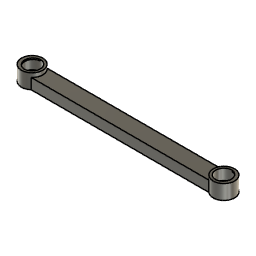
Sus_Arm_Prot_1 v1 (Autodesk Fusion 360 design; units mm, degrees)
Autodesk Fusion 360 part; units mm, degrees
sketch "Sketch1" plane through (0, 0, 0) normal (0, 0, 1) x (1, 0, 0)
  line L0 (0, 0) -> (32, 0)
  line L1 (32, 0) -> (32, -6)
  line L2 (32, -6) -> (0, -6)
  line L3 (0, -6) -> (0, 0)
  circle A0 centre (36.0053, -3) radius 4
  line L4 (32, 0) -> (33.3595, 0)
  line L5 (32, -6) -> (33.3595, -6)
  dimension "d1" = 32
  dimension "d2" = 6
  dimension "d3" = 8
  constraint horizontal L0
  constraint vertical L1
  constraint horizontal L2
  constraint vertical L3
  constraint coincident L0.start L3.end
  constraint coincident A0 L4.end
  constraint perpendicular L1 L4
  constraint coincident A0 L5.end
  constraint perpendicular L1 L5
  measures "d1" distance of L0.start L0.end
  measures "d2" distance of L0.start L2.end
  measures "d3" diameter of A0
extrude "Extrude1" add sketch "Sketch1" along normal blind 4 contours L0 L1 L2 L3 | L1 A0 L4 L5
extrude "Extrude2" add sketch "Sketch1" along normal blind 5.5 contours A0
hole "Hole1" at (36.0053, -3, 5.5) direction (0, 0, -1) diameter 6.2 depth 4 tip angle 180
sketch "Sketch2" plane through (0, 0, 5.5) normal (0, 0, 1) x (-1, 0, 0)
  circle A0 centre (-36.0053, 3) radius 3.1
  circle A1 centre (-36.0053, 3) radius 4
  arc A2 (-36.0053, 6.1) -> (-36.0053, -0.1) centre (-35.6842, 3) ccw
  constraint coincident A0 A2.start
  constraint coincident A0 A2.end
extrude "Extrude3" add sketch "Sketch2" against normal blind 0.5 contours A0 A2 picked at (-38.8883, 3.2291)
mirror "Mirror1" about plane through (0, -6, 0) normal (-1, 0, 0) of bodies 1 merged
